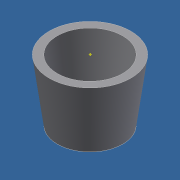
# Autodesk Inventor part: Lampignon_20x15
Saved by Autodesk Inventor 2018.2 (Build 222227000, 227)
## iProperties
Created: 2018-09-24
Part Number: Lampignon_20x15
Material: geeigneten Werkstoff auswählen !
Document SubType Name: Modeling
Designer: N.Grubert
Density: 0.001 g/cm^3
Appearance: Vorgabe
Fläche: 0 cm²
Gewicht: 0 g
Dateiname: P:\INVENTOR\Inventor 2018\Templates\ILT\Norm.ipt
Bez_eng: bolt
Bez_french: boulon
Author: N.Grubert
Autodesk Inventor part; units mm, degrees
ref_plane "YZ Plane" through (0, 0, 0) normal (1, 0, 0) x (0, 1, 0)
ref_plane "XZ Plane" through (0, 0, 0) normal (0, 1, 0) x (-1, 0, 0)
ref_plane "XY Plane" through (0, 0, 0) normal (0, 0, 1) x (1, 0, 0)
sketch "Skizze4" plane through (0, 0, 0) normal (1, 0, 0) x (0, 1, 0)
  line L0 (-2, 0) -> (12, 0) construction
  line L1 (0, -18) -> (0, 3) projected
  line L2 (10, 0) -> (8, -15)
  line L3 (6.0673, -14.4951) -> (8, 0)
  line L4 (6, -15) -> (8, 0)
  line L5 (10, 0) -> (8, 0)
  line L6 (6, -15) -> (8, -15)
  point P0 (0, 0)
  dimension "d6" = 20
  dimension "d7" = 12
  dimension "d8" = 2
  dimension "d9" = 15
  constraints: 10 end point, 2 collinear, 2 horizontal, 1 parallel
  measures "d6" diameter of L2.start L1
  measures "d7" diameter of L4.start L1
  measures "d8" distance of L4.start L2.end
  measures "d9" distance between parallel lines of L6 L0
revolve "Umdrehung1" add sketch "Skizze4" angle 360 about axis through (0, 0, -10) along (0, 0, 1)
